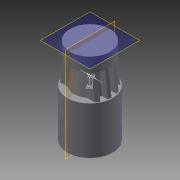
# Autodesk Inventor part: Engine Block
Saved by Autodesk Inventor 2015 (Build 190159000, 159)
## iProperties
Created: 2016-02-24
Part Number: Engine Block
Material: Generic
Document SubType Name: Modeling
Designer: Owner
Density: 1 g/cm^3
Appearance: Default
Author: Owner
Autodesk Inventor part; units mm, degrees
ref_plane "XZ Plane" through (0, 0, 0) normal (0, 1, 0) x (-1, 0, 0)
ref_plane "XY Plane" through (0, 0, 0) normal (0, 0, 1) x (1, 0, 0)
sketch "Sketch1" plane through (0, 0, 0) normal (0, 1, 0) x (-1, 0, 0)
  circle A0 centre (0, 0) radius 12.5095
  dimension "d0" = 25.019
  constraints: 1 centre point, 1 coincident
  measures "d0" diameter of A0
extrude "Extrusion1" add sketch "Sketch1" along normal blind 26.162
ref_plane "Work Plane1" through (0, 47.625, 0) normal (0, -1, 0) x (1, 0, 0)
sketch "Sketch2" plane through (0, 47.625, 0) normal (0, -1, 0) x (1, 0, 0)
  circle A0 centre (0, 0) radius 11.049
  dimension "d4" = 22.098
  constraints: 1 centre point, 1 coincident
  measures "d4" diameter of A0
extrude "Extrusion2" add sketch "Sketch2" along normal blind 7.62
sketch "Sketch4" plane through (0, 40.005, 0) normal (0, -1, 0) x (1, 0, 0)
  circle A0 centre (0, 0) radius 7.239
  dimension "d7" = 14.478
  constraints: 1 centre point, 1 coincident
  measures "d7" diameter of A0
sketch "Sketch5" plane through (0, 26.162, 0) normal (0, 1, 0) x (1, 0, 0)
  circle A0 centre (0, 0) radius 8.7122
  dimension "d8" = 17.4244
  constraints: 1 centre point, 1 coincident
  measures "d8" diameter of A0
loft "Loft1" add profiles "Sketch5", "Sketch4"
sketch "Sketch6" plane through (0, 40.005, 0) normal (0, -1, 0) x (1, 0, 0)
  circle A0 centre (0, 0) radius 10.414
  dimension "d13" = 20.828
  constraints: 1 centre point, 1 coincident
  measures "d13" diameter of A0
sketch "Sketch7" plane through (0, 26.162, 0) normal (0, 1, 0) x (1, 0, 0)
  circle A0 centre (0, 0) radius 11.8872
  dimension "d14" = 23.7744
  constraints: 1 centre point, 1 coincident
  measures "d14" diameter of A0
surface_loft "LoftSrf1"
sketch "Sketch8" plane through (0, 0, 0) normal (1, 0, 0) x (0, 1, 0)
  line L0 (47.625, -11.049) -> (40.005, -11.049) construction
  line L1 (40.005, -11.049) -> (40.005, -10.16) construction
  line L2 (40.005, 11.049) -> (40.005, -11.049) construction
  line L3 (40.005, -10.16) -> (26.162, -10.16)
  line L4 (26.162, -12.5095) -> (26.162, 12.5095) projected
  line L5 (40.005, -10.16) -> (40.005, -8.255)
  line L6 (40.005, -8.255) -> (26.162, -8.255)
  line L7 (40.005, -8.255) -> (40.005, -5.08) construction
  line L8 (40.005, -5.08) -> (26.162, -5.08)
  line L9 (26.162, -8.255) -> (26.162, -10.16)
  line L10 (40.005, -5.08) -> (40.005, -3.175)
  line L11 (40.005, -3.175) -> (26.162, -3.175)
  line L12 (26.162, -3.175) -> (26.162, -5.08)
  line L13 (40.005, 0) -> (40.005, 1.905)
  line L14 (40.005, 0) -> (26.162, 0)
  line L15 (26.162, 0) -> (26.162, 1.905)
  line L16 (40.005, 1.905) -> (26.162, 1.905)
  line L17 (40.005, 1.905) -> (40.005, 5.08) construction
  line L18 (40.005, 5.08) -> (26.162, 5.08)
  line L19 (26.162, 5.08) -> (26.162, 6.985)
  line L20 (26.162, 6.985) -> (40.005, 6.985)
  line L21 (40.005, 5.08) -> (40.005, 6.985)
  point P0 (0, 0)
  dimension "d19" = 0.889
  dimension "d20" = 1.905
  dimension "d21" = 3.175
  dimension "d22" = 1.905
  dimension "d23" = 1.905
  dimension "d24" = 3.175
  dimension "d25" = 1.905
  constraints: 38 end point, 6 horizontal, 3 vertical, 1 perpendicular, 1 point on line, 18 other
  measures "d19" distance of L1.start L1.end
  measures "d20" distance of L1.end L5.end
  measures "d21" distance of L5.end L7.end
  measures "d22" distance of L7.end L10.end
  measures "d23" distance of L13.start L13.end
  measures "d24" distance of L13.end L17.end
  measures "d25" distance of L18.end L19.end
extrude "Extrusion3" add sketch "Sketch8" along normal up to surface round surface about axis through (0, 26.162, 0) along (0, 1, 0) radius 11.8872 half angle -6.074668 far side no
mirror "Mirror1" about plane through (0, 0, 0) normal (1, 0, 0) of "Extrusion3"
sketch "Sketch10" plane through (0, 0, 0) normal (0, 0, 1) x (1, 0, 0)
  line L0 (-6.3487, 40.005) -> (6.3487, 40.005) projected
  line L1 (0, 40.005) -> (0, 26.162)
  line L2 (-5.2069, 26.162) -> (5.2069, 26.162) projected
  line L3 (0, 26.162) -> (1.27, 26.162)
  line L4 (1.27, 26.162) -> (1.27, 40.005)
  line L5 (0, 40.005) -> (1.27, 40.005)
  line L6 (0, 26.162) -> (-1.27, 26.162)
  line L7 (-1.27, 26.162) -> (-1.27, 40.005)
  line L8 (-1.27, 40.005) -> (0, 40.005)
  point P0 (0, 0)
  dimension "d28" = 1.27
  dimension "d29" = 1.27
  constraints: 14 end point, 4 point on line, 2 collinear, 2 midpoint, 2 perpendicular
  measures "d28" distance of L1.end L3.end
  measures "d29" distance of L1.end L6.end
body "Solid1"
body "Srf1"
